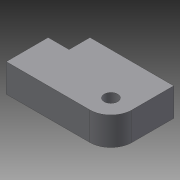
# Autodesk Inventor part: Carriage_Belt_Lock_Flap
Saved by Autodesk Inventor 2014 (Build 180170000, 170)
## iProperties
Created: 2014-09-19
Part Number: Carriage_Belt_Lock_Flap
Material: Generic
Document SubType Name: Modeling
Designer: ThatOtherGuy
Density: 1 g/cm^3
Appearance: Default
Author: ThatOtherGuy
Autodesk Inventor part; units mm, degrees
ref_plane "YZ Plane" through (0, 0, 0) normal (1, 0, 0) x (0, 1, 0)
ref_plane "XZ Plane" through (0, 0, 0) normal (0, 1, 0) x (-1, 0, 0)
ref_plane "XY Plane" through (0, 0, 0) normal (0, 0, 1) x (1, 0, 0)
sketch "Sketch1" plane through (0, 0, 0) normal (0, 0, 1) x (1, 0, 0)
  line L0 (0, 0) -> (25, 0)
  line L1 (25, 0) -> (25, 15)
  line L2 (25, 15) -> (5, 15)
  circle A0 centre (20, 5) radius 1.6
  line L3 (5, 10) -> (0, 10)
  line L4 (0, 10) -> (0, 0)
  line L5 (5, 10) -> (5, 15)
  dimension "d2" = 3.2
  dimension "d3" = 10
  dimension "d4" = 5
  dimension "d12" = 20
  dimension "d16" = 15
  dimension "d17" = 5
  dimension "d18" = 5
  constraints: 14 end point, 2 horizontal, 2 perpendicular, 1 centre point, 1 parallel
  measures "d2" diameter of A0
  measures "d3" distance of L0.start L3.end
  measures "d4" distance of L3.start L3.end
  measures "d12" distance between parallel lines of L1 L5
  measures "d16" distance between parallel lines of L0 L2
  measures "d17" distance from line of L0 A0.centre
  measures "d18" distance from line of A0.centre L1
extrude "Extrusion1" add sketch "Sketch1" along normal blind 6.731
fillet "Fillet1" radius 5 1 edges at (25, 0, 3.3655)
equation "\"d18\" = d17"
equation "\"d6\" = THICKB"
equation "\"THICKA\" = 3.175"
equation "\"THICKB\" = 6.731"
equation "\"THICKC\" = 12.7"
equation "\"BALLDIA\" = 12"
equation "\"MAGDIA\" = 9.5"
body "Solid1"
